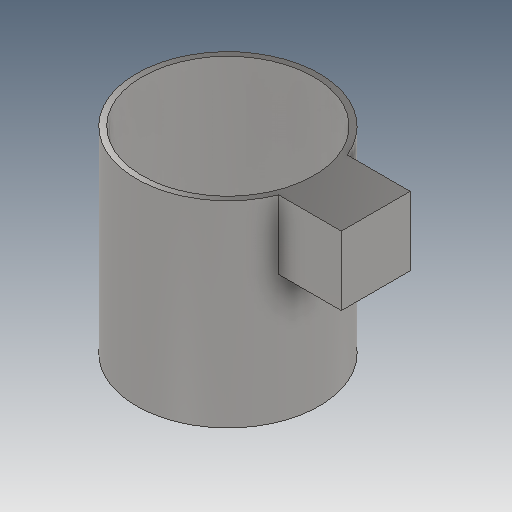
# Autodesk Inventor part: cock storage holder
Saved by Autodesk Inventor 2021 (Build 250183000, 183)
## iProperties
Created: 2021-06-18
Part Number: cock storage holder
Material: Stainless Steel
Document SubType Name: Modeling
Designer: user
Density: 8 g/cm^3
Appearance: Semi-Polished
Author: user
Autodesk Inventor part; units mm, degrees
ref_plane "YZ Plane" through (0, 0, 0) normal (1, 0, 0) x (0, 1, 0)
ref_plane "XZ Plane" through (0, 0, 0) normal (0, 1, 0) x (-1, 0, 0)
ref_plane "XY Plane" through (0, 0, 0) normal (0, 0, 1) x (1, 0, 0)
sketch "Sketch13" plane through (0, 0, 0) normal (0, 1, 0) x (-1, 0, 0)
  circle A0 centre (0, 0) radius 44.2659
  circle A1 centre (0, 0) radius 47.1927
  dimension "d24" = 88.5317
  constraints: 2 centre point, 2 coincident
  measures "d24" diameter of A0
extrude "Extrusion7" add sketch "Sketch13" along normal blind 101.6
sketch "Sketch14" plane through (0, 101.6, 0) normal (0, 1, 0) x (1, 0, 0)
  line L0 (43.6505, 17.9383) -> (76.2, 17.9383)
  line L1 (76.2, 17.9383) -> (76.2, -17.6217)
  line L2 (76.2, -17.6217) -> (43.7793, -17.6217)
  circle A0 centre (0, 0) radius 47.1927 projected
  arc A1 (43.7793, -17.6217) -> (43.6505, 17.9383) centre (0, 0) ccw
  dimension "d29" = 35.56
  constraints: 6 end point, 4 point on circle, 1 centre point, 1 horizontal, 1 parallel, 1 perpendicular
  measures "d29" distance of L0.end L1.end
extrude "Extrusion8" add sketch "Sketch14" against normal blind 35.56 contours L0 L1 L2 A0
body "Solid2"
